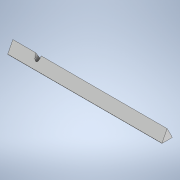
# Autodesk Inventor part: Grua Maya
Saved by Autodesk Inventor 2020 (Build 240168000, 168)
## iProperties
Created: 2019-10-05
Part Number: Grua Maya
Material: Genérico
Document SubType Name: Modeling
Designer: dasa1
Density: 1 g/cm^3
Appearance: Valor por defecto
Author: dasa1
Autodesk Inventor part; units mm, degrees
ref_plane "YZ Plane" through (0, 0, 0) normal (1, 0, 0) x (0, 1, 0)
ref_plane "XZ Plane" through (0, 0, 0) normal (0, 1, 0) x (-1, 0, 0)
ref_plane "XY Plane" through (0, 0, 0) normal (0, 0, 1) x (1, 0, 0)
sketch "Boceto1" plane through (0, 0, 0) normal (0, 1, 0) x (-1, 0, 0)
  line L0 (0, 0) -> (500, 0) construction
  line L1 (500, 0) -> (500, -200) construction
  line L2 (500, -200) -> (0, -200) construction
  line L3 (0, -200) -> (0, 0) construction
  line L4 (500, -200) -> (-2500, -200)
  line L5 (-2500, -200) -> (-2500, 0)
  line L6 (-2500, 0) -> (500, 0)
  line L7 (500, 0) -> (500, -200)
  dimension "d0" = 500
  dimension "d1" = 200
  dimension "d2" = 3000
  dimension "d3" = 200
  constraints: 16 end point, 4 parallel, 2 horizontal, 2 perpendicular
  measures "d0" distance of L1.end L2.end
  measures "d1" distance of L0.end L1.end
  measures "d2" distance of L5.end L6.end
  measures "d3" distance of L4.end L5.end
extrude "Extrusión1" add sketch "Boceto1" along normal blind 200
chamfer "Chaflán1" distance 100 angle 63 2 edges at (1000, 200, 0) (1000, 200, -200) measured on face at (1000, 200, -0.5) measured on face at (1000, 200, -199.5)
sketch "Boceto2" plane through (0, 0, 0) normal (0, -1, 0) x (1, 0, 0)
  line L0 (-500, -200) -> (-500, 0) construction
  line L1 (-500, 0) -> (0, 0) construction
  line L2 (0, 0) -> (0, -100) construction
  line L3 (0, -100) -> (-500, -100) construction
  line L4 (-500, -100) -> (-500, 0) construction
  circle A0 centre (0, -100) radius 50
  constraints: 8 end point, 2 parallel, 1 centre point, 1 coincident, 1 horizontal, 1 perpendicular
hole "Agujero1" at (0, 0, -100) direction (0, 1, 0) diameter 100 end through all
